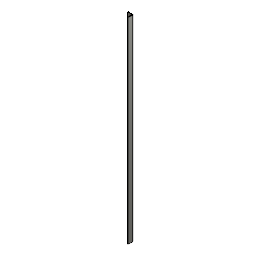
30part (Autodesk Fusion 360 design; units mm, degrees)
Autodesk Fusion 360 part; units mm, degrees
sketch "Sketch1" plane through (0, 0, 0) normal (0, 1, 0) x (1, 0, 0)
  line L0 (60, 51) -> (75, 51)
  line L1 (75, 51) -> (75, 49.5)
  line L2 (75, 49.5) -> (60, 49.5)
  line L3 (60, 49.5) -> (60, 51)
  line L4 (73.5, 51) -> (75, 51)
  line L5 (75, 51) -> (75, 36)
  line L6 (75, 36) -> (73.5, 36)
  line L7 (73.5, 36) -> (73.5, 51)
  dimension "d14" = 15
  dimension "d15" = 1.5
  dimension "d16" = 15
  dimension "d17" = 1.5
  constraint horizontal L0
  constraint vertical L1
  constraint horizontal L2
  constraint vertical L3
  constraint horizontal L4
  constraint vertical L5
  constraint horizontal L6
  constraint vertical L7
  measures "d14" distance of L0.start L0.end
  measures "d15" distance of L0.start L2.end
  measures "d16" distance of L4.start L6.end
  measures "d17" distance of L0.end L4.start
extrude "Extrude1" add sketch "Sketch1" along normal blind 550
